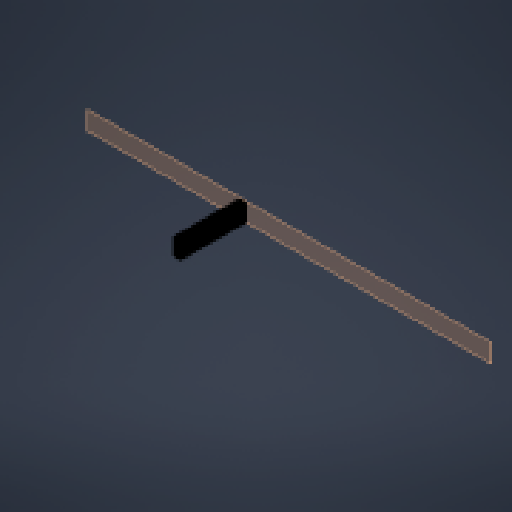
# Autodesk Inventor part: 2x4x16
Saved by Autodesk Inventor 2027 (Build 310192000, 192)
## iProperties
Created: 2026-08-07
Part Number: 2x4x16
Material: Generic
Document SubType Name: Modeling
Designer: lucas
Density: 1 g/cm^3
Appearance: Default
Author: lucas
Autodesk Inventor part; units mm, degrees
ref_plane "YZ Plane" through (0, 0, 0) normal (1, 0, 0) x (0, 1, 0)
ref_plane "XZ Plane" through (0, 0, 0) normal (0, 1, 0) x (-1, 0, 0)
ref_plane "XY Plane" through (0, 0, 0) normal (0, 0, 1) x (1, 0, 0)
ref_plane "Work Plane1" through (0, 0, 0) normal (0, 0, 1) x (1, 0, 0)
sketch "Sketch1" plane through (0, 0, 0) normal (0, 0, 1) x (1, 0, 0)
  line L0 (-1117.6, -50.8) -> (1117.6, -50.8) projected
  line L1 (1117.6, 50.8) -> (-1117.6, 50.8) projected
  line L2 (-304.8, 50.8) -> (-254, 50.8)
  line L3 (-254, 50.8) -> (-254, -50.8)
  line L4 (-254, -50.8) -> (-304.8, -50.8)
  line L5 (-304.8, -50.8) -> (-304.8, 50.8)
  point P0 (0, 0)
  point P1 (-482.6, -152.4)
  dimension "d0" = 50.8
  dimension "d1" = 177.8
  constraints: 8 end point, 2 parallel, 2 point on line, 1 horizontal, 1 perpendicular, 1 other
  measures "d0" distance between parallel lines of L3 L5
  measures "d1" distance from line of point (-482.6, -152.4) L5
extrude "Extrusion1" add sketch "Sketch1" along normal blind 406.4
body "Solid1"
